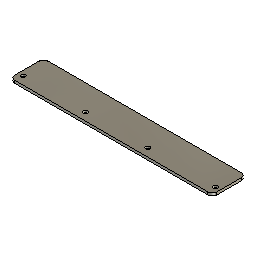
Weight (Autodesk Fusion 360 design; units mm, degrees)
Autodesk Fusion 360 part; units mm, degrees
sketch "Weight" plane through (0, 0, 0) normal (0, 0, 1) x (1, 0, 0)
  circle A0 centre (107.0661, -8.5483) radius 1.235
  circle A1 centre (-109.5839, -8.5496) radius 1.235
  line L0 (-109.5839, -8.5496) -> (-108.3489, -8.5502)
  circle A2 centre (-39.4339, -8.5498) radius 1.235
  circle A3 centre (30.7061, -8.5641) radius 1.235
  line L1 (29.4711, -8.5635) -> (30.7061, -8.5641)
  line L2 (-115.0339, 14.7839) -> (-115.0339, -12.7161)
  line L3 (107.6661, -17.7161) -> (-110.0339, -17.7161)
  line L4 (112.6661, 14.7839) -> (112.6661, -12.7161)
  line L5 (107.6661, 19.7839) -> (-110.0339, 19.7839)
  line L6 (-115.0339, -8.5498) -> (112.6661, -8.5498)
  arc A4 (-110.0339, 19.7839) -> (-115.0339, 14.7839) centre (-110.0339, 14.7839) ccw
  arc A5 (-115.0339, -12.7161) -> (-110.0339, -17.7161) centre (-110.0339, -12.7161) ccw
  arc A6 (107.6661, -17.7161) -> (112.6661, -12.7161) centre (107.6661, -12.7161) ccw
  arc A7 (112.6661, 14.7839) -> (107.6661, 19.7839) centre (107.6661, 14.7839) ccw
  dimension "d10" = 2.47
  dimension "d11" = 2.47
  dimension "d20" = 2.47
  dimension "d21" = 2.47
  dimension "d27" = 227.7
  dimension "d28" = 37.5
  dimension "d29" = 5.45
  dimension "d30" = 75.6
  dimension "d31" = 145.74
  dimension "d32" = 222.1
  dimension "d58" = 5
  dimension "d59" = 5
  constraint coincident A1.centre L0.start
  constraint coincident A3.centre L1.end
  constraint coincident A3 L1.start
  constraint coincident A1 L0.end
  constraint coincident L2 L6.start
  constraint coincident L4 L6.end
  constraint perpendicular L4 L6
  constraint tangent L2 A4
  constraint tangent L5 A4
  constraint tangent L2 A5
  constraint tangent L3 A5
  constraint equal A4 A5
  constraint tangent L3 A6
  constraint tangent L4 A6
  constraint equal A4 A6
  constraint tangent L5 A7
  constraint tangent L4 A7
  measures "d10" diameter of A0
  measures "d11" diameter of A1
  measures "d20" diameter of A2
  measures "d21" diameter of A3
  measures "d27" distance of L2 L4
  measures "d28" distance of L3 L5
  measures "d29" distance of A1.centre L6.start
  measures "d30" distance of A2.centre L6.start
  measures "d31" distance of A3.centre L6.start
  measures "d32" horizontal distance of A0.centre L6.start
  measures "d58" radius of A4
  measures "d59" radius of A7
extrude "ExMain Body" add sketch "Weight" along normal blind 3 contours A0 A1 A2 A3 L2 L3 L4 L6 A5 A6 | A0 A1 A2 A3 L2 L4 L5 L6 A4 A7
sketch "Sketch2" plane through (0, 0, 3) normal (0, 0, 1) x (-1, 0, 0)
  line L0 (-112.6661, 12.7161) -> (-112.6661, -14.7839)
  line L1 (115.0339, -14.7839) -> (115.0339, 12.7161)
  line L2 (110.0339, 17.7161) -> (-107.6661, 17.7161)
  line L3 (91.5212, 0) -> (50, 0) construction
  line L4 (50, 0) -> (50, -14.5112) construction
  line L5 (50, -14.5112) -> (91.5212, -14.5112) construction
  line L6 (91.5212, -14.5112) -> (91.5212, 0) construction
  arc A0 (115.0339, 12.7161) -> (110.0339, 17.7161) centre (110.0339, 12.7161) ccw
  arc A1 (-107.6661, 17.7161) -> (-112.6661, 12.7161) centre (-107.6661, 12.7161) ccw
  circle A2 centre (39.4339, 8.5498) radius 1.235
  circle A3 centre (-30.7061, 8.5641) radius 1.235
  circle A4 centre (109.5839, 8.5496) radius 1.235
  circle A5 centre (-107.0661, 8.5483) radius 1.235
  arc A6 (-112.6661, -14.7839) -> (-107.6661, -19.7839) centre (-107.6661, -14.7839) ccw
  line L7 (-107.6661, -19.7839) -> (110.0339, -19.7839)
  arc A7 (110.0339, -19.7839) -> (115.0339, -14.7839) centre (110.0339, -14.7839) ccw
  dimension "d35" = 10
hole "Hole2" at (-39.4339, -8.5498, 3) direction (0, 0, -1) diameter 2 depth 9 tip angle 180 countersink diameter 4.8 countersink angle 90
hole "Hole3" at (-109.5839, -8.5496, 3) direction (0, 0, -1) diameter 2 depth 9 tip angle 180 countersink diameter 4.8 countersink angle 90
hole "Hole4" at (30.7061, -8.5641, 3) direction (0, 0, -1) diameter 2 depth 9 tip angle 180 countersink diameter 4.8 countersink angle 90
hole "Hole5" at (107.0661, -8.5483, 3) direction (0, 0, -1) diameter 2 depth 9 tip angle 180 countersink diameter 4.8 countersink angle 90
equation "d10 = d11"
equation "d20 = d11"
equation "d21 = d11"
